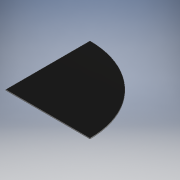
# Autodesk Inventor part: Black Glass Corner Piece
Saved by Autodesk Inventor 2016 (Build 200138000, 138)
## iProperties
Created: 2015-11-19
Part Number: Black Glass Corner Piece
Material: 玻璃
Document SubType Name: Modeling
Designer: Shawn Shi Feng
Density: 2.18 g/cm^3
Appearance: 清晰
Author: Shawn Shi Feng
Autodesk Inventor part; units mm, degrees
ref_plane "YZ Plane" through (0, 0, 0) normal (1, 0, 0) x (0, 1, 0)
ref_plane "XZ Plane" through (0, 0, 0) normal (0, 1, 0) x (-1, 0, 0)
ref_plane "XY Plane" through (0, 0, 0) normal (0, 0, 1) x (1, 0, 0)
sketch "草图1" plane through (0, 0, 0) normal (0, 0, 1) x (1, 0, 0)
  line L0 (-188.7661, 285.9116) -> (-188.7661, -214.0884)
  line L1 (-188.7661, -214.0884) -> (311.2339, -214.0884)
  arc A0 (311.2339, -214.0884) -> (-188.7661, 285.9116) centre (-188.7661, -214.0884) ccw
  point P0 (0, 0)
  dimension "d0" = 500
  dimension "d1" = 500
  dimension "d2" = 90
  dimension "d3" = 500
  constraints: 4 end point, 2 point on circle, 1 centre point, 1 vertical
  measures "d0" distance of L0.start L0.end
  measures "d1" distance of L0.end L1.end
  measures "d2" angle of L1 L0
  measures "d3" radius of A0
extrude "拉伸1" add sketch "草图1" along normal blind 5
